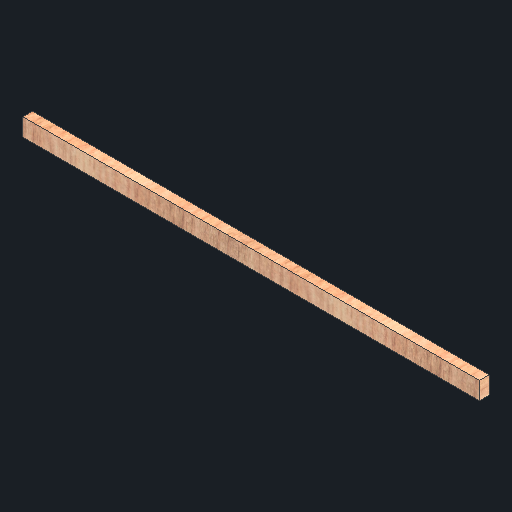
# Autodesk Inventor part: BASE_FRONT,BACK_TREBUCHET
Saved by Autodesk Inventor 2026.2 (Build 302298010, 298A)
## iProperties
Created: 2026-02-18
Part Number: BASE_FRONT,BACK_TREBUCHET
Material: Wood (Birch)
Document SubType Name: Modeling
Designer: 4aida
Density: 0.55 g/cm^3
Appearance: Birch - Natural Polished
Mass: 41.2445 g
Surface Area: 246.673 cm^2
Volume: 74.99 cm^3
Author: 4aida
Autodesk Inventor part; units mm, degrees
ref_plane "YZ Plane" through (0, 0, 0) normal (1, 0, 0) x (0, 1, 0)
ref_plane "XZ Plane" through (0, 0, 0) normal (0, 1, 0) x (-1, 0, 0)
ref_plane "XY Plane" through (0, 0, 0) normal (0, 0, 1) x (1, 0, 0)
sketch "Sketch1" plane through (0, 0, 0) normal (0, 0, 1) x (1, 0, 0)
  line L0 (225.425, -8.7312) -> (-225.425, -8.7312)
  line L1 (-225.425, 8.7312) -> (225.425, 8.7312)
  line L2 (-225.425, -8.7312) -> (225.425, 8.7312) construction
  line L3 (0, 0) -> (0, 8.7313) construction
  line L4 (-225.425, -8.7312) -> (-225.425, 0)
  line L5 (-225.425, 0) -> (-225.425, 8.7312)
  line L6 (225.425, -8.7312) -> (225.425, 0)
  line L7 (225.425, 0) -> (225.425, 8.7312)
  dimension "d6" = 225.425
  dimension "d14" = 17.4625
  constraints: 16 end point, 2 midpoint, 2 parallel, 2 perpendicular, 2 symmetric about line, 1 horizontal, 1 horizontal alignment, 1 vertical
  measures "d6" distance from line of L3.start L4
  measures "d14" distance between parallel lines of L1 L0
extrude "Extrusion1" add sketch "Sketch1" along normal blind 9.525
body "Solid1"
